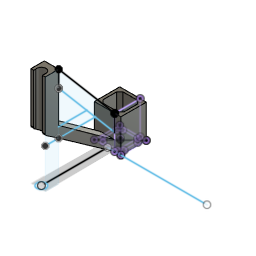
VerticalTransducerHolder (Autodesk Fusion 360 design; units mm, degrees)
Autodesk Fusion 360 part; units mm, degrees
sketch "Sketch1" plane through (0, 0, 0) normal (0, 1, 0) x (1, 0, 0)
sketch "Sketch2" plane through (0, 0, 0) normal (1, 0, 0) x (0, 0, -1)
sketch "Sketch3" plane through (0, 0, 0) normal (0, 1, 0) x (1, 0, 0)
sketch "Sketch4" plane through (0, 0, 0) normal (0, 1, 0) x (1, 0, 0)
  line L0 (1.5, 7) -> (-5, 7)
  line L1 (8, -10) -> (10.5, -7.5)
  line L2 (10.5, -1.5) -> (10.5, -7.5)
  line L3 (-7.5, -1.5) -> (-7.5, -7.5)
  line L4 (1.5, 7) -> (8, 7)
  line L5 (10.5, -1.5) -> (10.5, -7.5)
  line L6 (1.5, -10) -> (8, -10)
  line L7 (10.5, -10) -> (-7.5, 7) construction
  line L8 (1.5, -10) -> (8, -10)
  line L9 (10.5, 7) -> (10.5, -10)
  line L10 (8, 7) -> (10.5, 4.5)
  line L11 (-7.5, -1.5) -> (-7.5, 4.5)
  line L12 (10.5, -1.5) -> (10.5, 4.5)
  line L13 (-7.5, 7) -> (10.5, 7)
  line L14 (-7.5, -7.5) -> (-5, -10)
  line L15 (-7.5, -10) -> (10.5, 7) construction
  line L16 (-7.5, 4.5) -> (-5, 7)
  line L17 (-7.5, -10) -> (-7.5, 7)
  line L18 (10.5, -10) -> (-7.5, -10)
  line L19 (1.5, -10) -> (-5, -10)
  line L20 (13.5, 10) -> (-10.5, 10)
  line L21 (-10.5, 10) -> (-10.5, -13)
  line L22 (-10.5, -13) -> (13.5, -13)
  line L23 (13.5, -13) -> (13.5, 10)
  line L24 (13.5, 10) -> (-10.5, -13) construction
  line L25 (-10.5, 10) -> (13.5, -13) construction
  line L26 (1.5, -10.5) -> (-5.2071, -10.5)
  line L27 (-8, -7.7071) -> (-5.2071, -10.5)
  line L28 (-8, -1.5) -> (-8, -7.7071)
  line L29 (-8, -1.5) -> (-8, 4.7071)
  line L30 (-8, 4.7071) -> (-5.2071, 7.5)
  line L31 (1.5, 7.5) -> (-5.2071, 7.5)
  line L32 (1.5, 7.5) -> (8.2071, 7.5)
  line L33 (8.2071, 7.5) -> (11, 4.7071)
  line L34 (11, -1.5) -> (11, 4.7071)
  line L35 (11, -1.5) -> (11, -7.7071)
  line L36 (8.2071, -10.5) -> (11, -7.7071)
  line L37 (1.5, -10.5) -> (8.2071, -10.5)
  point P0 (1.5, -1.5)
  point P1 (1.5, -1.5)
  point P2 (1.5, -1.5)
  dimension "d1" = 18
  dimension "d2" = 17
  dimension "d3" = 6
  dimension "d4" = 6
  dimension "d5" = 6.5
  dimension "d6" = 6.5
  dimension "d7" = 6
  dimension "d8" = 6
  dimension "d9" = 6.5
  dimension "d10" = 6.5
  dimension "d11" = 6.5
  dimension "d12" = 6
  dimension "d13" = 24
  dimension "d14" = 23
  dimension "d15" = -0.5
  constraint horizontal L18
  constraint perpendicular L17 L18
  constraint parallel L13 L18
  constraint parallel L9 L17
  constraint coincident P2 L7
  constraint coincident P2 L15
  constraint coincident P2 P1
  constraint midpoint L3.start L17
  constraint parallel L11 L17
  constraint parallel L3 L17
  constraint midpoint L6.start L18
  constraint parallel L8 L18
  constraint parallel L18 L19
  constraint midpoint L2.start L9
  constraint parallel L9 L12
  constraint coincident L1.end L9
  constraint midpoint L0.start L13
  constraint parallel L4 L13
  constraint parallel L0 L13
  constraint parallel L6 L18
  constraint parallel L2 L5
  constraint horizontal L20
  constraint perpendicular L20 L21
  constraint parallel L20 L22
  constraint parallel L21 L23
  constraint coincident L24 P2
  constraint coincident L25 P2
  measures "d1" distance of L7.end L9.start
  measures "d2" distance of L15.start L7.end
  measures "d3" distance of L3.start L11.end
  measures "d4" distance of L3.start L3.end
  measures "d5" distance of L1.start L6.start
  measures "d6" distance of L6.start L14.end
  measures "d7" distance of L2.start L10.end
  measures "d8" distance of L1.end L2.start
  measures "d9" distance of L0.start L4.end
  measures "d10" distance of L0.start L0.end
  measures "d11" distance of L1.start L6.start
  measures "d12" distance of L1.end L2.start
  measures "d13" distance of L21.end L22.end
  measures "d14" distance of L20.end L21.end
extrude "Extrude1" add sketch "Sketch4" along normal blind 30 contours L13 L17 L30 | L9 L13 L33 | L17 L18 L27 | L9 L18 L36 | L20 L21 L22 L23 makes body 1
sketch "Sketch5" plane through (0, 0, 0) normal (0, -1, 0) x (1, 0, 0)
  line L0 (-8, -4.7071) -> (-8, 7.7071)
  line L1 (-8, 7.7071) -> (-5.2071, 10.5)
  line L2 (-5.2071, 10.5) -> (8.2071, 10.5)
  line L3 (8.2071, 10.5) -> (11, 7.7071)
  line L4 (11, 7.7071) -> (11, -4.7071)
  line L5 (11, -4.7071) -> (8.2071, -7.5)
  line L6 (8.2071, -7.5) -> (-5.2071, -7.5)
  line L7 (-5.2071, -7.5) -> (-8, -4.7071)
  line L8 (13.5, -10) -> (13.5, 13)
  line L9 (13.5, 13) -> (-10.5, 13)
  line L10 (-10.5, 13) -> (-10.5, -10)
  line L11 (-10.5, -10) -> (13.5, -10)
  line L12 (-10.5, 13) -> (13.5, -10)
  line L13 (13.5, 13) -> (-10.5, -10)
  point P0 (1.5, 1.5)
  constraint coincident L9.end L10.start
  constraint coincident L8.start L11.end
  constraint coincident L8.end L9.start
  constraint coincident L10.end L11.start
  constraint midpoint L13 P0
sketch "Sketch6" plane through (0, 0, 0) normal (0, -1, 0) x (1, 0, 0)
  line L0 (-8, -4.7071) -> (-8, 7.7071)
  line L1 (-8, 7.7071) -> (-5.2071, 10.5)
  line L2 (-5.2071, 10.5) -> (8.2071, 10.5)
  line L3 (8.2071, 10.5) -> (11, 7.7071)
  line L4 (11, 7.7071) -> (11, -4.7071)
  line L5 (11, -4.7071) -> (8.2071, -7.5)
  line L6 (8.2071, -7.5) -> (-5.2071, -7.5)
  line L7 (-5.2071, -7.5) -> (-8, -4.7071)
  line L8 (13.5, -10) -> (13.5, 13)
  line L9 (13.5, 13) -> (-10.5, 13)
  line L10 (-10.5, 13) -> (-10.5, -10)
  line L11 (-10.5, -10) -> (13.5, -10)
  line L12 (1.5, 13) -> (1.5, 73)
  dimension "d18" = 60
  constraint midpoint L9 L12.start
  constraint perpendicular L9 L12
  measures "d18" distance of L12.start L12.end
ref_plane "WorkPlane1" through (1.5, 0, 43) normal (0, -1, 0) x (0, 0, 1)
sketch "Sketch7" plane through (1.5, 0, 43) normal (0, -1, 0) x (0, 0, 1)
  line L0 (-30, 0) -> (-30, -90)
  dimension "d20" = 90
  constraint vertical L0
  measures "d20" distance of L0.start L0.end
ref_plane "WorkPlane2" through (46.5, 0, 13) normal (0, 0, -1) x (1, 0, 0)
sketch "Sketch25" plane through (1.5, 0, 43) normal (0, -1, 0) x (1, 0, 0)
  circle A0 centre (0, 30) radius 4.075
  dimension "d74" = 8.15
  measures "d74" diameter of A0
sketch "Sketch26" plane through (0, 0, 0) normal (0, 1, 0) x (1, 0, 0)
  circle A0 centre (1.5, -73) radius 4.075
  line L0 (8, -74) -> (-5, -74)
  line L1 (-5, -74) -> (-5, -63.85)
  line L2 (-5, -63.85) -> (8, -63.85)
  line L3 (8, -63.85) -> (8, -74)
  line L4 (8, -74) -> (-5, -63.85) construction
  line L5 (-5, -74) -> (8, -63.85) construction
  point P0 (1.5, -68.925)
  constraint horizontal L0
  constraint perpendicular L0 L1
  constraint parallel L0 L2
  constraint parallel L1 L3
  constraint coincident L4 P0
  constraint coincident L5 P0
  constraint coincident A0 P0
extrude "Extrude18" add sketch "Sketch26" along normal blind 90 separate body contours A0 L0 L1 L2 L3 makes body 2
extrude "Extrude19" add 2 faces at (-3.3003, 60, 74) (7.1501, 30, 74) along direction (0, 0, 1) blind 2 on bodies 2 bodies 2
sketch "Sketch27" plane through (8, 0, 0) normal (1, 0, 0) x (0, 0, -1)
  line L0 (-76, 0) -> (-63.85, 0)
  line L1 (-63.85, 0) -> (-63.85, 90)
  line L2 (-63.85, 90) -> (-76, 90)
  line L3 (-76, 90) -> (-76, 0)
  line L4 (-13, 0) -> (10, 0)
  line L5 (10, 0) -> (10, 30)
  line L6 (10, 30) -> (-13, 30)
  line L7 (-13, 30) -> (-13, 0)
  line L8 (-63.85, 90) -> (-13, 30)
  line L9 (-63.85, 90) -> (-63.85, 75)
  line L10 (-13, 30) -> (-13, 15)
  line L11 (-63.85, 75.12) -> (-13, 15)
  line L12 (-63.85, 45) -> (-38.425, 45.06)
  line L13 (-63.85, 35.9416) -> (-30.7126, 35.9416)
  line L14 (-63.85, 35.9416) -> (-76, 35.9416)
  constraint coincident L1.end L2.start
  constraint coincident L6.end L7.start
  constraint coincident L1 L9.end
  constraint midpoint L7 L10.end
  constraint midpoint L1 L12.start
  constraint midpoint L11 L12.end
  constraint coincident L1 L13.start
  constraint coincident L11 L13.end
  constraint perpendicular L1 L13
  constraint coincident L3 L14.end
  constraint perpendicular L3 L14
extrude "Extrude20" cut sketch "Sketch27" against normal blind 30 contours L0 L1 L3 L14 bodies 2
sketch "Sketch32" plane through (-5, 0, 0) normal (-1, 0, 0) x (0, 0, 1)
  line L0 (63.85, 35.9416) -> (76, 35.9416)
  line L1 (76, 35.9416) -> (76, 90)
  line L2 (76, 90) -> (63.85, 90)
  line L3 (63.85, 90) -> (63.85, 35.9416)
  line L4 (-10, 0) -> (13, 0)
  line L5 (13, 0) -> (13, 30)
  line L6 (13, 30) -> (-10, 30)
  line L7 (-10, 30) -> (-10, 0)
  line L8 (63.85, 35.9416) -> (13, 0)
  line L9 (63.85, 35.9416) -> (63.85, 45.9416)
  line L10 (63.85, 45.9416) -> (13, 9.2584)
  dimension "d108" = 10
  constraint coincident L0.start L3.end
  constraint coincident L4.end L5.start
  constraint coincident L3 L9.end
  constraint coincident L5 L10.end
  measures "d108" distance of L0.start L9.end
extrude "Extrude28" add sketch "Sketch32" against normal blind 13 contours L3 L5 L8 L9 L10 bodies 1 2
sketch "Sketch33" plane through (8, 0, 0) normal (1, 0, 0) x (0, 0, -1)
  line L0 (-63.85, 35.9416) -> (-83, 49)
  line L1 (-63.85, 35.9416) -> (-76, 35.9416)
  line L2 (-76, 90) -> (-76, 0)
  line L3 (-63.85, 35.9416) -> (-13, 0)
  constraint coincident L0.start L1.start
extrude "Extrude29" cut sketch "Sketch33" against normal blind 38 bodies 1
fillet "Fillet4" radius 2 2 edges at (-3.7252, 44.2267, 76) (6.7252, 44.2267, 76) on bodies 1
equation "d13 = 18.000 mm + 6 mm"
equation "d14 = 17.000 mm + 6 mm"
